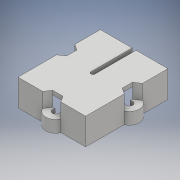
# Autodesk Inventor part: Protector
Saved by Autodesk Inventor 2017 (Build 210142000, 142)
## iProperties
Created: 2018-03-30
Part Number: Protector
Material: Generic
Document SubType Name: Modeling
Designer: andrew
Density: 1 g/cm^3
Appearance: Default
Author: andrew
Autodesk Inventor part; units mm, degrees
note: some values were not read from the file. Chosen so that the rebuilt part matches the saved one: sketch regions of "Extrusion2".
ref_plane "YZ Plane" through (0, 0, 0) normal (1, 0, 0) x (0, 1, 0)
ref_plane "XZ Plane" through (0, 0, 0) normal (0, 1, 0) x (-1, 0, 0)
ref_plane "XY Plane" through (0, 0, 0) normal (0, 0, 1) x (1, 0, 0)
sketch "Sketch1" plane through (0, 0, 0) normal (0, 0, 1) x (1, 0, 0)
  arc A0 (-6, -5.5) -> (-5.5, -6) centre (-5.5, -5.5) ccw
  line L0 (-6, -5.5) -> (-6, 5.5)
  arc A1 (-5.5, 6) -> (-6, 5.5) centre (-5.5, 5.5) ccw
  line L1 (-5.5, 6) -> (5.5, 6)
  arc A2 (6, 5.5) -> (5.5, 6) centre (5.5, 5.5) ccw
  line L2 (6, 5.5) -> (6, -5.5)
  arc A3 (5.5, -6) -> (6, -5.5) centre (5.5, -5.5) ccw
  line L3 (5.5, -6) -> (-5.5, -6)
  circle A4 centre (-7.5, 3.5) radius 0.375
  circle A5 centre (7.5, 3.5) radius 0.85
  circle A6 centre (0, -7.5) radius 0.375
  arc A7 (2.2913, -7) -> (0.9165, -7.9) centre (2.2913, -8.5) ccw
  line L4 (2.2913, -7) -> (7, -7)
  line L5 (7, -7) -> (7, 1.2087)
  arc A8 (7.9, 2.5835) -> (7, 1.2087) centre (8.5, 1.2087) ccw
  arc A9 (7.9, 2.5835) -> (7.9, 4.4165) centre (7.5, 3.5) ccw
  arc A10 (7, 5.7913) -> (7.9, 4.4165) centre (8.5, 5.7913) ccw
  line L6 (7, 5.7913) -> (7, 6.5)
  line L7 (-7, 6) -> (-7, 5.7913)
  arc A11 (-7.9, 4.4165) -> (-7, 5.7913) centre (-8.5, 5.7913) ccw
  arc A12 (-7.9, 4.4165) -> (-7.9, 2.5835) centre (-7.5, 3.5) ccw
  arc A13 (-7, 1.2087) -> (-7.9, 2.5835) centre (-8.5, 1.2087) ccw
  line L8 (-7, 1.2087) -> (-7, -7)
  line L9 (-7, -7) -> (-2.2913, -7)
  arc A14 (-0.9165, -7.9) -> (-2.2913, -7) centre (-2.2913, -8.5) ccw
  arc A15 (-0.9165, -7.9) -> (0.9165, -7.9) centre (0, -7.5) ccw
  line L10 (-7, 6) -> (-7, 10.7)
  line L11 (7, 6.5) -> (7, 10.7)
  line L12 (-7, 10.7) -> (7, 10.7)
  line L13 (-7.5, -7.5) -> (-7.5, 1.2087)
  arc A16 (-7.5, 1.2087) -> (-8.1, 2.1252) centre (-8.5, 1.2087) ccw
  arc A17 (-8.1, 4.8748) -> (-8.1, 2.1252) centre (-7.5, 3.5) ccw
  arc A18 (-8.1, 4.8748) -> (-7.5, 5.7913) centre (-8.5, 5.7913) ccw
  line L14 (-7.5, 5.7913) -> (-7.5, 6)
  line L15 (-7.5, 6) -> (-7.5, 11.2)
  line L16 (-7.5, 11.2) -> (7.5, 11.2)
  line L17 (7.5, 11.2) -> (7.5, 6.5)
  line L18 (7.5, 6.5) -> (7.5, 5.7913)
  arc A19 (7.5, 5.7913) -> (8.1, 4.8748) centre (8.5, 5.7913) ccw
  arc A20 (8.1, 2.1252) -> (8.1, 4.8748) centre (7.5, 3.5) ccw
  arc A21 (8.1, 2.1252) -> (7.5, 1.2087) centre (8.5, 1.2087) ccw
  line L19 (7.5, 1.2087) -> (7.5, -7.5)
  line L20 (7.5, -7.5) -> (2.2913, -7.5)
  arc A22 (2.2913, -7.5) -> (1.3748, -8.1) centre (2.2913, -8.5) ccw
  arc A23 (-1.3748, -8.1) -> (1.3748, -8.1) centre (0, -7.5) ccw
  arc A24 (-1.3748, -8.1) -> (-2.2913, -7.5) centre (-2.2913, -8.5) ccw
  line L21 (-2.2913, -7.5) -> (-7.5, -7.5)
  line L22 (-8.5, 12.2) -> (-8.5, 6)
  line L23 (-8.5, 6) -> (-8.5, 5.7913)
  arc A25 (-8.5, 5.7913) -> (-8.5, 1.2087) centre (-7.5, 3.5) ccw
  line L24 (-8.5, 1.2087) -> (-8.5, -8.5)
  line L25 (-8.5, -8.5) -> (-2.2913, -8.5)
  arc A26 (-2.2913, -8.5) -> (2.2913, -8.5) centre (0, -7.5) ccw
  line L26 (2.2913, -8.5) -> (8.5, -8.5)
  line L27 (8.5, -8.5) -> (8.5, 1.2087)
  arc A27 (8.5, 1.2087) -> (8.5, 5.7913) centre (7.5, 3.5) ccw
  line L28 (8.5, 5.7913) -> (8.5, 6.5)
  line L29 (8.5, 6.5) -> (8.5, 12.2)
  line L30 (8.5, 12.2) -> (-8.5, 12.2)
  point P0 (0, 0)
  point P1 (0, 0)
  dimension "d1" = 0.5
  dimension "d2" = 1
  dimension "d30" = 1.7
  constraints: 62 end point, 50 point on circle, 28 centre point, 1 horizontal, 28 other
  measures "d1" distance between parallel lines of L8 L13
  measures "d2" distance between parallel lines of L15 L22
  measures "d30" diameter of A5
extrude "Extrusion1" add sketch "Sketch1" along normal blind 2 contours L30 L29 L28 A27 L27 L26 A26 L25 L24 A25 L23 L22
sketch "Sketch3" plane through (0, 0, 2) normal (0, 0, 1) x (1, 0, 0)
  circle A0 centre (0, -7.5) radius 0.85
  arc A1 (-0.9165, -7.9) -> (0.9165, -7.9) centre (0, -7.5) ccw
  arc A2 (2.2913, -7) -> (0.9165, -7.9) centre (2.2913, -8.5) ccw
  arc A3 (7.9, 2.5835) -> (7, 1.2087) centre (8.5, 1.2087) ccw
  circle A4 centre (7.5, 3.5) radius 0.85
  arc A5 (7.9, 2.5835) -> (7.9, 4.4165) centre (7.5, 3.5) ccw
  arc A6 (6, 5.5) -> (5.5, 6) centre (5.5, 5.5) ccw
  line L0 (7, 5.7913) -> (7, 6.5)
  arc A7 (7, 5.7913) -> (7.9, 4.4165) centre (8.5, 5.7913) ccw
  circle A8 centre (-7.5, 3.5) radius 0.85
  arc A9 (-7, 1.2089) -> (-7.8999, 2.5836) centre (-8.5, 1.2089) ccw
  arc A10 (-7.8999, 4.4166) -> (-7.8999, 2.5836) centre (-7.4998, 3.5001) ccw
  line L1 (-7, 6) -> (-7, 5.7913)
  arc A11 (-7.8999, 4.4166) -> (-7, 5.7913) centre (-8.5, 5.7913) ccw
  arc A12 (-0.9165, -7.9) -> (-2.2913, -7) centre (-2.2913, -8.5) ccw
  arc A13 (5.5, -6) -> (6, -5.5) centre (5.5, -5.5) ccw
  line L2 (2.2913, -7) -> (7, -7)
  arc A14 (-6, -5.5) -> (-5.5, -6) centre (-5.5, -5.5) ccw
  line L3 (-7, -7) -> (-2.2913, -7)
  line L4 (7, -7) -> (7, 1.2087)
  line L5 (5.5, -6) -> (-5.5, -6)
  line L6 (6, 5.5) -> (6, -5.5)
  line L7 (-5.5, 6) -> (5.5, 6)
  line L8 (-6, -5.5) -> (-6, 5.5)
  arc A15 (-5.5, 6) -> (-6, 5.5) centre (-5.5, 5.5) ccw
  line L9 (-7, 1.2089) -> (-7, -7)
  line L10 (-7, 6) -> (-7, 10.7)
  line L11 (7, 6.5) -> (7, 10.7)
  line L12 (-7, 10.7) -> (7, 10.7)
  line L13 (-7.5, -7.5) -> (-7.5, 1.2089)
  arc A16 (-7.5, 1.2089) -> (-8.0999, 2.1254) centre (-8.5, 1.2089) ccw
  arc A17 (-8.0999, 4.8748) -> (-8.0999, 2.1254) centre (-7.4998, 3.5001) ccw
  arc A18 (-8.0999, 4.8748) -> (-7.5, 5.7913) centre (-8.5, 5.7913) ccw
  line L14 (-7.5, 5.7913) -> (-7.5, 6)
  line L15 (-7.5, 6) -> (-7.5, 11.2)
  line L16 (-7.5, 11.2) -> (7.5, 11.2)
  line L17 (7.5, 11.2) -> (7.5, 6.5)
  line L18 (7.5, 6.5) -> (7.5, 5.7913)
  arc A19 (7.5, 5.7913) -> (8.1, 4.8748) centre (8.5, 5.7913) ccw
  arc A20 (8.1, 2.1252) -> (8.1, 4.8748) centre (7.5, 3.5) ccw
  arc A21 (8.1, 2.1252) -> (7.5, 1.2087) centre (8.5, 1.2087) ccw
  line L19 (7.5, 1.2087) -> (7.5, -7.5)
  line L20 (7.5, -7.5) -> (2.2913, -7.5)
  arc A22 (2.2913, -7.5) -> (1.3748, -8.1) centre (2.2913, -8.5) ccw
  arc A23 (-1.3748, -8.1) -> (1.3748, -8.1) centre (0, -7.5) ccw
  arc A24 (-1.3748, -8.1) -> (-2.2913, -7.5) centre (-2.2913, -8.5) ccw
  line L21 (-2.2913, -7.5) -> (-7.5, -7.5)
  line L22 (-8.5, 12.2) -> (-8.5, 6)
  line L23 (-8.5, 6) -> (-8.5, 5.7913)
  arc A25 (-8.5, 5.7913) -> (-8.5, 1.2089) centre (-7.4998, 3.5001) ccw
  line L24 (-8.5, 1.2089) -> (-8.5, -8.5)
  line L25 (-8.5, -8.5) -> (-2.2913, -8.5)
  arc A26 (-2.2913, -8.5) -> (2.2913, -8.5) centre (0, -7.5) ccw
  line L26 (2.2913, -8.5) -> (8.5, -8.5)
  line L27 (8.5, -8.5) -> (8.5, 1.2087)
  arc A27 (8.5, 1.2087) -> (8.5, 5.7913) centre (7.5, 3.5) ccw
  line L28 (8.5, 5.7913) -> (8.5, 6.5)
  line L29 (8.5, 6.5) -> (8.5, 12.2)
  line L30 (8.5, 12.2) -> (-8.5, 12.2)
  line L31 (-7.5, 11.2) -> (-7.5, 5.7913) projected
  line L32 (-7.5, 5.7913) -> (-7, 5.7913)
  line L33 (-7.5, 1.2089) -> (-7, 1.2089)
  line L34 (7, 5.7913) -> (7.5, 5.7913)
  line L35 (7.5, 1.2087) -> (7.5, -7.5) projected
  line L36 (7, 1.2087) -> (7.5, 1.2087)
  line L37 (7, 5.7913) -> (7, 1.2087)
  line L38 (-7, 1.2089) -> (-7, 5.7913)
  line L39 (-2.2913, -7) -> (-2.2913, -7.5)
  line L40 (2.2913, -7) -> (2.2913, -7.5)
  line L41 (2.2913, -7) -> (-2.2913, -7)
  point P0 (0, 0)
  point P1 (0, 0)
  point P2 (0, 0)
  dimension "d5" = 0.5
  dimension "d6" = 1
  dimension "d31" = 1.7
  dimension "d34" = 1.7
  dimension "d35" = 1.7
  constraints: 80 end point, 50 point on circle, 28 centre point, 5 parallel, 2 horizontal, 2 perpendicular, 1 vertical, 28 other
  measures "d5" distance between parallel lines of L9 L13
  measures "d6" distance between parallel lines of L15 L22
  measures "d31" diameter of A4
  measures "d34" diameter of A8
  measures "d35" diameter of A0
extrude "Extrusion2" add sketch "Sketch3" along normal blind 1 contours A0 L41 A2 A1 A12 | L40 A22 A23 A24 L39 A12 A1 A2 | L37 A4 A7 A5 A3 | A3 A5 A7 L34 A19 A20 A21 L36 | L33 A16 A17 A18 L32 A11 A10 A9 | A9 A10 A11 L38 A8 | L30 L29 L28 A27 L27 L26 A26 L25 L24 A25 L23 L22
sketch "Sketch4" plane through (0, 0, 3) normal (0, 0, 1) x (1, 0, 0)
  arc A0 (6, 5.5) -> (5.5, 6) centre (5.5, 5.5) ccw construction
  line L0 (7, 5.7913) -> (7, 6.5) construction
  line L1 (-7, 6) -> (-7, 5.7913) construction
  arc A1 (5.5, -6) -> (6, -5.5) centre (5.5, -5.5) ccw construction
  line L2 (2.2913, -7) -> (7, -7) construction
  arc A2 (-6, -5.5) -> (-5.5, -6) centre (-5.5, -5.5) ccw construction
  line L3 (-7, -7) -> (-2.2913, -7) construction
  line L4 (7, -7) -> (7, 1.2087) construction
  line L5 (5.5, -6) -> (-5.5, -6) construction
  line L6 (6, 5.5) -> (6, -5.5) construction
  line L7 (-5.5, 6) -> (5.5, 6) construction
  line L8 (-6, -5.5) -> (-6, 5.5) construction
  arc A3 (-5.5, 6) -> (-6, 5.5) centre (-5.5, 5.5) ccw construction
  line L9 (-7, 1.2089) -> (-7, -7) construction
  line L10 (-7, 6) -> (-7, 10.7) construction
  line L11 (7, 6.5) -> (7, 10.7) construction
  line L12 (-7, 10.7) -> (7, 10.7) construction
  line L13 (-7.5, 5.7913) -> (-7.5, 6) construction
  line L14 (-7.5, 6.9093) -> (-7.5, 11.2) construction
  line L15 (-7.5, 11.2) -> (7.5, 11.2) construction
  line L16 (7.5, 6.5) -> (7.5, 6) construction
  line L17 (-8.5, 12.2) -> (-8.5, 6) construction
  line L18 (-8.5, 6) -> (-8.5, 5.7913) construction
  line L19 (-8.5, 1.2087) -> (-8.5, -8.5) construction
  line L20 (-8.5, -8.5) -> (-2.2913, -8.5) construction
  line L21 (2.2913, -8.5) -> (8.5, -8.5) construction
  line L22 (8.5, -8.5) -> (8.5, 1.2087) construction
  line L23 (8.5, 5.7913) -> (8.5, 6.5) construction
  line L24 (8.5, 6.5) -> (8.5, 12.2) construction
  line L25 (8.5, 12.2) -> (-8.5, 12.2) construction
  line L26 (-7, 4.7913) -> (-8.5, 5.7913) construction
  line L27 (-7, 2.2087) -> (-8.5, 1.2087) construction
  line L28 (-7.5, -7.5) -> (-7.5, 0.0907) construction
  line L29 (-7.5, 1) -> (-7.5, 1.2087) construction
  line L30 (0, 3.5) -> (0, 6) construction
  line L31 (7, 4.7913) -> (8.5, 5.7913) construction
  line L32 (7, 2.2087) -> (8.5, 1.2087) construction
  line L33 (7.5, 11.2) -> (7.5, 10.7) construction
  line L34 (7.5, 6.9093) -> (7.5, 6.5) construction
  line L35 (7.5, 1.2087) -> (7.5, 1) construction
  line L36 (7.5, 0.0907) -> (7.5, -7.5) construction
  circle A4 centre (-1.1674, -14.5937) radius 0.375 construction
  line L37 (-2.4587, -14.0937) -> (-3.4587, -15.5937) construction
  line L38 (0.1239, -14.0937) -> (1.1239, -15.5937) construction
  line L39 (-1.2913, -7) -> (-2.2913, -8.5) construction
  line L40 (1.2913, -7) -> (2.2913, -8.5) construction
  line L41 (-2.2913, -7.5) -> (-2.5, -7.5) construction
  line L42 (-3.4093, -7.5) -> (-7.5, -7.5) construction
  line L43 (7.5, -7.5) -> (3.4093, -7.5) construction
  line L44 (2.5, -7.5) -> (2.2913, -7.5) construction
  line L45 (-2.2913, -7) -> (-1.2913, -7) construction
  line L46 (-7, 2.2087) -> (-7, 1.2089) construction
  line L47 (7, 5.7913) -> (7, 4.7913) construction
  line L48 (1.2913, -7) -> (7, -7) construction
  line L49 (7, 2.2087) -> (7, 1.2087) construction
  line L50 (-7, 5.7913) -> (-7, 4.7913) construction
  line L51 (8.5, 12.2) -> (-8.5, 12.2) projected
  line L52 (-8.5, 12.2) -> (-8.5, 5.7913)
  line L53 (-7, 4.7913) -> (-8.5, 5.7913)
  line L54 (-7, 4.7913) -> (-7, 10.7)
  line L55 (-7, 10.7) -> (7, 10.7)
  line L56 (7, 10.7) -> (7, 4.7913)
  line L57 (7, 4.7913) -> (8.5, 5.7913)
  line L58 (8.5, 5.7913) -> (8.5, 12.2)
  line L59 (8.5, 12.2) -> (-8.5, 12.2)
  line L60 (-7, 2.2087) -> (-8.5, 1.2087)
  line L61 (-8.5, 1.2087) -> (-8.5, -8.5)
  line L62 (-8.5, -8.5) -> (-2.2913, -8.5)
  line L63 (-7, -7) -> (-7, 2.2087)
  line L64 (-7, 5.7913) -> (-7, 1.2089) projected
  line L65 (1.2913, -7) -> (2.2913, -8.5)
  line L66 (2.2913, -8.5) -> (8.5, -8.5)
  line L67 (8.5, -8.5) -> (8.5, 1.2087)
  line L68 (8.5, 1.2087) -> (7, 2.2087)
  line L69 (7, 2.2087) -> (7, -7)
  line L70 (-8.5, -8.5) -> (-2.2913, -8.5) projected
  line L71 (-2.2913, -8.5) -> (-1.2913, -7)
  line L72 (-1.2913, -7) -> (-7, -7)
  line L73 (1.2913, -7) -> (7, -7)
  line L74 (-2.2913, -7) -> (2.2913, -7) projected
  point P0 (0, 0)
  point P1 (0, 0)
  point P2 (0, 0)
  dimension "d10" = 1
  constraints: 142 end point, 8 point on circle, 6 collinear, 6 perpendicular, 5 centre point, 5 vertical, 4 symmetric about line, 2 horizontal, 2 parallel, 2 point on line, 1 midpoint
  measures "d10" distance between parallel lines of L14 L17
extrude "Extrusion3" add sketch "Sketch4" along normal blind 2.7
sketch "Sketch5" plane through (0, 0, 5.7) normal (0, 0, 1) x (1, 0, 0)
  line L0 (-7, 10.7) -> (7, 10.7) projected
  line L1 (7, 10.7) -> (7, 4.7913) projected
  line L2 (7, 4.7913) -> (8.5, 5.7913) projected
  line L3 (8.5, 5.7913) -> (8.5, 12.2) projected
  line L4 (8.5, 12.2) -> (-8.5, 12.2) projected
  line L5 (-8.5, 12.2) -> (-8.5, 5.7913) projected
  line L6 (-8.5, 5.7913) -> (-7, 4.7913) projected
  line L7 (-7, 4.7913) -> (-7, 10.7) projected
  line L8 (7, 2.2087) -> (7, -7) projected
  line L9 (7, -7) -> (1.2913, -7) projected
  line L10 (1.2913, -7) -> (2.2913, -8.5) projected
  line L11 (2.2913, -8.5) -> (8.5, -8.5) projected
  line L12 (8.5, -8.5) -> (8.5, 1.2087) projected
  line L13 (8.5, 1.2087) -> (7, 2.2087) projected
  line L14 (-7, -7) -> (-7, 2.2087) projected
  line L15 (-7, 2.2087) -> (-8.5, 1.2087) projected
  line L16 (-8.5, 1.2087) -> (-8.5, -8.5) projected
  line L17 (-8.5, -8.5) -> (-2.2913, -8.5) projected
  line L18 (-2.2913, -8.5) -> (-1.2913, -7) projected
  line L19 (-1.2913, -7) -> (-7, -7) projected
  line L20 (-1.2913, -7) -> (1.2913, -7) projected
  line L21 (7, 2.2087) -> (7, 4.7913) projected
  line L22 (-7, 4.7913) -> (-7, 2.2087) projected
  line L23 (-7, 10.7) -> (7, 10.7) construction
  line L24 (0, 10.7) -> (7, 10.7) construction
  line L25 (7, 10.7) -> (7, -7) construction
  line L26 (7, -7) -> (0, -7) construction
  line L27 (0, -7) -> (0, 10.7) construction
  circle A0 centre (0, 1.85) radius 0.5
  point P0 (0, 0)
  dimension "d16" = 1
  constraints: 8 end point, 2 midpoint, 2 parallel, 1 centre point, 1 horizontal, 1 perpendicular
  measures "d16" diameter of A0
extrude "Extrusion4" add sketch "Sketch5" along normal blind 1
sketch "Sketch14" plane through (0, 0, 6.7) normal (0, 0, 1) x (1, 0, 0)
  circle A0 centre (0, 1.85) radius 0.5 projected
  line L0 (0.5, 1.85) -> (-0.5, 1.85)
  line L1 (-0.5, 1.85) -> (-0.5, 13.3555)
  line L2 (-0.5, 13.3555) -> (0.5, 13.3555)
  line L3 (0.5, 13.3555) -> (0.5, 1.85)
  point P0 (0, 0)
  constraints: 8 end point, 2 parallel, 1 horizontal, 1 horizontal alignment, 1 perpendicular, 1 other
extrude "Extrusion6" cut sketch "Sketch14" against normal blind 10 contours L0 A0 | A0 L1 L2 L3 picked at (0.1248, 1.9605)
body "Solid1"
